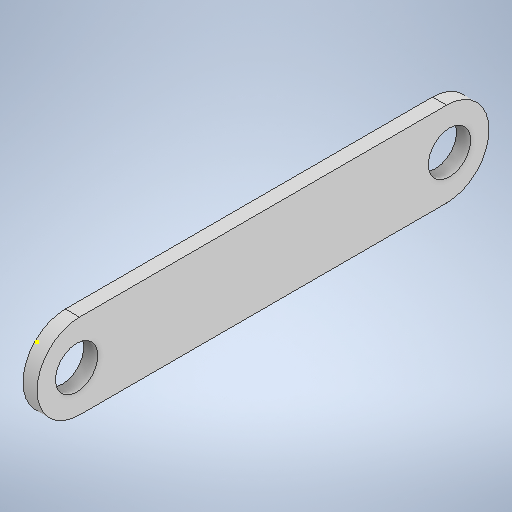
# Autodesk Inventor part: Acoplador
Saved by Autodesk Inventor 2025.2 (Build 292293000, 293)
## iProperties
Created: 2026-09-08
Part Number: Acoplador
Material: Generic
Document SubType Name: Sheet Metal
Designer: dguar
Density: 1 g/cm^3
Sheet Metal Rule: Default_mm
Appearance: Default
Author: dguar
Autodesk Inventor part; units mm, degrees
ref_plane "YZ Plane" through (0, 0, 0) normal (1, 0, 0) x (0, 1, 0)
ref_plane "XZ Plane" through (0, 0, 0) normal (0, 1, 0) x (-1, 0, 0)
ref_plane "XY Plane" through (0, 0, 0) normal (0, 0, 1) x (1, 0, 0)
sketch "Sketch1" plane through (0, 0, 0) normal (1, 0, 0) x (0, 1, 0)
  line L0 (0, 0) -> (-30, 0)
  line L1 (-30, 0) -> (-30, -160)
  line L2 (-30, -160) -> (0, -160)
  line L3 (0, -160) -> (0, 0)
  circle A0 centre (-15, -14) radius 7.5
  circle A1 centre (-15, -146) radius 7.5
  dimension "d0" = 30
  dimension "d1" = 160
  dimension "d3" = 15
  dimension "d5" = 15
  constraints: 8 end point, 2 centre point, 2 parallel, 1 horizontal, 1 perpendicular
  measures "d0" distance of L2.end L1.end
  measures "d1" distance of L1.end L0.end
  measures "d3" diameter of A0
  measures "d5" diameter of A1
extrude "Extrusion1" add sketch "Sketch1" along normal blind 5
sketch "Sketch2" plane through (5, 0, 0) normal (1, 0, 0) x (0, 0, -1)
  circle A0 centre (14, -15) radius 7.5 projected
  arc A1 (14, 0) -> (14, -30) centre (14, -15) ccw
  line L0 (0, -30) -> (160, -30) projected
  circle A2 centre (146, -15) radius 7.5 projected
  arc A3 (146, -30) -> (146, 0) centre (146, -15) ccw
  line L1 (146, -30) -> (161, -30)
  line L2 (161, -30) -> (161, 0)
  line L3 (161, 0) -> (146, 0)
  line L4 (14, 0) -> (-1, 0)
  line L5 (-1, 0) -> (-1, -30)
  line L6 (-1, -30) -> (14, -30)
  point P0 (0, 0)
  point P1 (-1, -15)
  point P2 (161, -15)
  constraints: 12 end point, 4 perpendicular, 4 point on circle, 4 tangent, 3 point on line, 2 centre point, 2 coincident, 1 horizontal
extrude "Extrusion2" cut sketch "Sketch2" along normal blind 10 contours A3 L3 L2 | A3 L2 L1 L0 | A1 L0 L6 L5 | A1 L5 L4
fillet "Fillet1" radius 15 4 edges at (2.5, 0, 0) (2.5, -30, 0) (2.5, 0, -160) (2.5, -30, -160)
sketch "Sketch3" plane through (5, 0, 0) normal (1, 0, 0) x (0, 0, -1)
  point P0 (0, 0)
equation "\"BendRadius\" = Thickness"
equation "\"BendReliefWidth\" = Thickness"
equation "\"BendReliefDepth\" = 0.5 * Thickness"
equation "\"CornerReliefSize\" = 4 * Thickness"
equation "\"MinimumRemnant\" = 2 * Thickness"
equation "\"TransitionRadius\" = BendRadius"
equation "\"JacobiRadiusSize\" = BendRadius"
equation "\"GapSize\" = Thickness"
equation "\"Thickness\" = 0.5"
body "Solid1"
